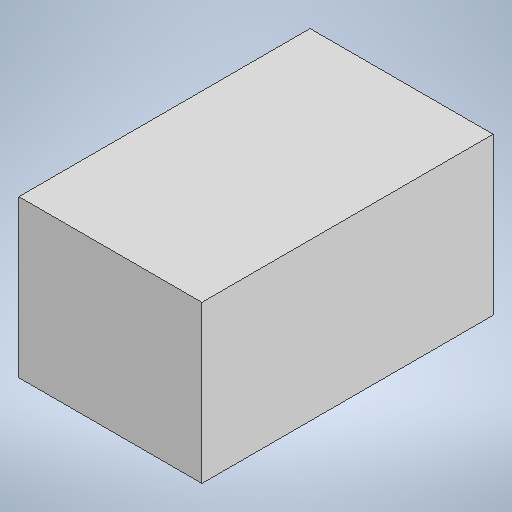
# Autodesk Inventor part: Контроллер EZrun max5
Saved by Autodesk Inventor 2025.1 (Build 291241000, 241)
## iProperties
Created: 2025-04-07
Part Number: Контроллер EZrun max5
Material: Типовые
Document SubType Name: Modeling
Designer: Root
Density: 1 g/cm^3
Appearance: По умолчанию
Author: Root
Autodesk Inventor part; units mm, degrees
ref_plane "YZ Plane" through (0, 0, 0) normal (1, 0, 0) x (0, 1, 0)
ref_plane "XZ Plane" through (0, 0, 0) normal (0, 1, 0) x (-1, 0, 0)
ref_plane "XY Plane" through (0, 0, 0) normal (0, 0, 1) x (1, 0, 0)
sketch "Эскиз1" plane through (0, 0, 0) normal (0, 1, 0) x (-1, 0, 0)
  line L0 (-29.7, -47.25) -> (29.7, -47.25)
  line L1 (29.7, -47.25) -> (29.7, 47.25)
  line L2 (29.7, 47.25) -> (-29.7, 47.25)
  line L3 (-29.7, 47.25) -> (-29.7, -47.25)
  line L4 (-29.7, -47.25) -> (29.7, 47.25) construction
  line L5 (29.7, -47.25) -> (-29.7, 47.25) construction
  point P0 (0, 0)
  dimension "d0" = 59.4
  dimension "d1" = 94.5
  constraints: 12 end point, 2 midpoint, 2 parallel, 1 horizontal, 1 perpendicular
  measures "d0" distance of L2.end L1.end
  measures "d1" distance of L1.end L0.end
extrude "Выдавливание1" add sketch "Эскиз1" along normal blind 50.9
